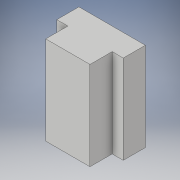
# Autodesk Inventor part: Back slide plate and side bar attatchment
Saved by Autodesk Inventor 2017 (Build 210142000, 142)
## iProperties
Created: 2017-10-11
Part Number: Back slide plate and side bar attatchment
Material: Generic
Document SubType Name: Modeling
Designer: Kenneth
Density: 1 g/cm^3
Appearance: Default
Author: Kenneth
Autodesk Inventor part; units mm, degrees
ref_plane "YZ Plane" through (0, 0, 0) normal (1, 0, 0) x (0, 1, 0)
ref_plane "XZ Plane" through (0, 0, 0) normal (0, 1, 0) x (-1, 0, 0)
ref_plane "XY Plane" through (0, 0, 0) normal (0, 0, 1) x (1, 0, 0)
sketch "Sketch2" plane through (0, 0, 0) normal (0, 0, 1) x (1, 0, 0)
  point P0 (0, 0)
sketch "Sketch3" plane through (0, 0, 0) normal (0, 0, 1) x (1, 0, 0)
  line L0 (-19.05, -25.4) -> (19.05, -25.4)
  line L1 (19.05, -25.4) -> (19.05, 25.4)
  line L2 (19.05, 25.4) -> (-19.05, 25.4)
  line L3 (-19.05, 25.4) -> (-19.05, -25.4)
  line L4 (-19.05, -25.4) -> (19.05, 25.4) construction
  line L5 (19.05, -25.4) -> (-19.05, 25.4) construction
  point P0 (0, 0)
  dimension "d4" = 50.8
  dimension "d5" = 38.1
  constraints: 12 end point, 2 midpoint, 2 parallel, 1 horizontal, 1 perpendicular
  measures "d4" distance of L0.end L1.end
  measures "d5" distance of L1.end L2.end
extrude "Extrusion2" add sketch "Sketch3" along normal blind 12.7
sketch "Sketch4" plane through (0, 0, 12.7) normal (0, 0, 1) x (1, 0, 0)
  line L0 (19.05, 25.4) -> (-19.05, 25.4) projected
  line L1 (12.7, -25.4) -> (-12.7, -25.4)
  line L2 (-12.7, -25.4) -> (-12.7, 25.4)
  line L3 (-12.7, 25.4) -> (12.7, 25.4)
  line L4 (12.7, 25.4) -> (12.7, -25.4)
  line L5 (12.7, -25.4) -> (-12.7, 25.4) construction
  line L6 (-12.7, -25.4) -> (12.7, 25.4) construction
  point P0 (0, 0)
  dimension "d8" = 25.4
  constraints: 12 end point, 2 midpoint, 2 parallel, 1 horizontal, 1 perpendicular, 1 point on line
  measures "d8" distance of L1.start L1.end
extrude "Extrusion3" add sketch "Sketch4" along normal blind 12.7
body "Solid1"
